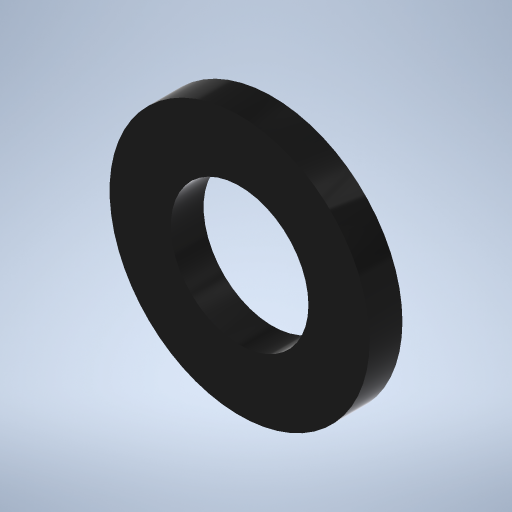
# Autodesk Inventor part: WASHER,FLAT,Z, M8
Saved by Autodesk Inventor 2024.2 (Build 282272000, 272)
## iProperties
Manager: 100-14500
Category: _
Material: Acetal Resin, Black
Document SubType Name: Modeling
Created: 2013-02-13
Designer: keithl , Keith
Manufacturer: Standard
Standards Organization: Custom
Checked By: 1JWML
Engr Approved By: R
User Status: Released
Description: WASHER, FLAT, Z, M8
Mass: 1.70713 g
Surface Area: 4.01253 cm^2
Volume: 0.217193 cm^3
Density: 1.425 g/cm^3
Mfg Approved By: Justin.Coates
Part Number: WASHER,FLAT,Z, M8
Appearance: Smooth - Black
Control State: 0
Master: False
Checked Out: False
Shininess: 64.0
Angle Display Precision: 2
Document Length Units: 11269
Document Angle Units: 11279
Document Time Units: 11290
Document Mass Units: 11283
Document Length Units Precision: 3
Document Angle Units Precision: 2
CN_SERVICEABLE: _
FIRST_DESCRIPTION: WASHER, FLAT, Z, M8
PTC_WM_ITERATION: 5
PTC_WM_ORGANIZATION_ID: CLWC
PTC_WM_LIFECYCLE: CLWC_CAD_LC
CN_MASS: 0.001707
CL_runCount: 1
FinishProperty: ToBeSet
SECOND_DESCRIPTION: _
THIRD_DESCRIPTION: _
CUSTOMERNUMBER: _
Density: 0.0
Volumn: 0.0
Area: 0.0
PropertySet Name: Model Information
Subject: _
Revision Number: 1
Author: -
Keywords: -
Autodesk Inventor part; units mm, degrees
ref_plane "YZ Plane" through (0, 0, 0) normal (1, 0, 0) x (0, 1, 0)
ref_plane "XZ Plane" through (0, 0, 0) normal (0, 1, 0) x (-1, 0, 0)
ref_plane "XY Plane" through (0, 0, 0) normal (0, 0, 1) x (1, 0, 0)
sketch "Sketch1" plane through (0, 0, 0) normal (0, 0, 1) x (1, 0, 0)
  circle A0 centre (0, 0) radius 7.9375
  circle A1 centre (0, 0) radius 4.2
  dimension "d0" = 15.875
  dimension "d1" = 8.4
  constraints: 2 centre point, 2 coincident
  measures "d0" diameter of A0
  measures "d1" diameter of A1
extrude "Extrusion1" add sketch "Sketch1" along normal blind 2
body "Solid1"
